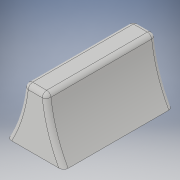
# Autodesk Inventor part: DoubleSliderCap
Saved by Autodesk Inventor 2018.3 (Build 223284000, 284)
## iProperties
Created: 2019-03-27
Part Number: DoubleSliderCap
Material: Generic
Document SubType Name: Modeling
Designer: matth
Density: 1 g/cm^3
Appearance: Default
Author: matth
Autodesk Inventor part; units mm, degrees
ref_plane "YZ Plane" through (0, 0, 0) normal (1, 0, 0) x (0, 1, 0)
ref_plane "XZ Plane" through (0, 0, 0) normal (0, 1, 0) x (-1, 0, 0)
ref_plane "XY Plane" through (0, 0, 0) normal (0, 0, 1) x (1, 0, 0)
sketch "Sketch1" plane through (0, 0, 0) normal (0, 0, 1) x (1, 0, 0)
  line L0 (-4.7637, 0) -> (8.2363, 0)
  line L1 (8.2363, 0) -> (8.2363, 13)
  line L2 (8.2363, 13) -> (-4.7637, 13)
  line L3 (-4.7637, 13) -> (-4.7637, 0)
  arc A0 (-4.7637, 0) -> (-0.7637, 13) centre (-33.6274, 15.9965) ccw
  arc A1 (4.2363, 13) -> (8.2363, 0) centre (37.1, 15.9965) ccw
  point P0 (0, 0)
  dimension "d0" = 13
  dimension "d1" = 13
  dimension "d2" = 4
  dimension "d3" = 4
  dimension "d4" = 33
  dimension "d5" = 33
  constraints: 8 end point, 4 point on circle, 3 perpendicular, 2 centre point, 2 point on line, 1 horizontal
  measures "d0" distance of L0.start L0.end
  measures "d1" distance of L0.end L1.end
  measures "d2" distance from line of L3 A0.end
  measures "d3" distance of L1.end A1.start
  measures "d4" radius of A0
  measures "d5" radius of A1
extrude "Extrusion1" add sketch "Sketch1" along normal blind 25 contours A0 L2 A1 L0
sketch "Sketch2" plane through (-4.7637, 0, 0) normal (0, -1, 0) x (1, 0, 0)
  line L0 (4, 21.2125) -> (9.2, 21.2125)
  line L1 (9.2, 21.2125) -> (9.2, 19.8125)
  line L2 (9.2, 19.8125) -> (4, 19.8125)
  line L3 (4, 19.8125) -> (4, 21.2125)
  line L4 (4, 5.1875) -> (9.2, 5.1875)
  line L5 (9.2, 5.1875) -> (9.2, 3.7875)
  line L6 (9.2, 3.7875) -> (4, 3.7875)
  line L7 (4, 3.7875) -> (4, 5.1875)
  line L8 (0, 0) -> (0, 25) projected
  line L9 (0, 25) -> (13, 25) projected
  point P0 (4.7637, 0)
  dimension "d8" = 5.2
  dimension "d9" = 4
  dimension "d10" = 1.4
  dimension "d11" = 1.4
  dimension "d12" = 17.425
  dimension "d13" = 3.7875
  constraints: 16 end point, 4 parallel, 2 horizontal, 2 perpendicular, 2 point on line
  measures "d8" distance between parallel lines of L1 L3
  measures "d9" distance between parallel lines of L8 L3
  measures "d10" distance between parallel lines of L0 L2
  measures "d11" distance of L6.end L4.start
  measures "d12" distance between parallel lines of L6 L0
  measures "d13" distance between parallel lines of L9 L0
extrude "Extrusion2" cut sketch "Sketch2" against normal blind 2
sketch "Sketch3" plane through (-4.7637, 2, 0) normal (0, -1, 0) x (1, 0, 0)
  line L0 (4.4, 21.2125) -> (8.8, 21.2125)
  line L1 (8.8, 21.2125) -> (8.8, 19.8125)
  line L2 (8.8, 19.8125) -> (4.4, 19.8125)
  line L3 (4.4, 19.8125) -> (4.4, 21.2125)
  line L4 (4, 19.8125) -> (4, 21.2125) projected
  line L5 (9.2, 21.2125) -> (9.2, 19.8125) projected
  line L6 (4, 21.2125) -> (9.2, 21.2125) projected
  line L7 (9.2, 19.8125) -> (4, 19.8125) projected
  line L8 (4, 5.1875) -> (9.2, 5.1875) projected
  line L9 (4, 3.7875) -> (4, 5.1875) projected
  line L10 (9.2, 3.7875) -> (4, 3.7875) projected
  line L11 (9.2, 5.1875) -> (9.2, 3.7875) projected
  line L12 (9.2, 3.7875) -> (4, 3.7875) projected
  line L13 (4.4, 5.1875) -> (8.8, 5.1875)
  line L14 (8.8, 5.1875) -> (8.8, 3.7875)
  line L15 (8.8, 3.7875) -> (4.4, 3.7875)
  line L16 (4.4, 3.7875) -> (4.4, 5.1875)
  point P0 (4.7637, 0)
  dimension "d16" = 0.4
  dimension "d17" = 0.4
  dimension "d18" = 0
  dimension "d19" = 0
  constraints: 16 end point, 4 parallel, 2 horizontal, 2 perpendicular, 2 point on line
  measures "d16" distance between parallel lines of L4 L3
  measures "d17" distance between parallel lines of L5 L1
  measures "d18" distance between parallel lines of L6 L0
  measures "d19" distance between parallel lines of L7 L2
extrude "Extrusion3" cut sketch "Sketch3" against normal blind 10 contours L0 L1 L2 L3 | L8 L14 L10 L16
fillet "Fillet1" radius 1 8 edges at (4.2363, 13, 12.5) (1.7363, 13, 25) (-0.7637, 13, 12.5) (1.7363, 13, 0) (5.5593, 6.2917, 25) (-2.0867, 6.2917, 25) (5.5593, 6.2917, 0) (-2.0867, 6.2917, 0)
body "Solid1"
